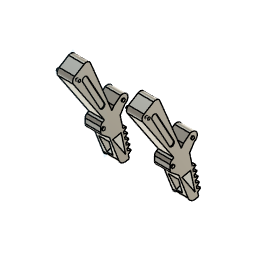
JAW FINAL v2 (Autodesk Fusion 360 design; units mm, degrees)
Autodesk Fusion 360 part; units mm, degrees
sketch "Sketch1" plane through (0, 0, 0) normal (1, 0, 0) x (0, 1, 0)
  line L0 (308.6071, 26.1218) -> (329.0653, 38.6702)
  line L1 (329.0653, 38.6702) -> (356.1703, -26.9523)
  line L2 (364.0358, -80.7741) -> (365.4972, -87.6198)
  line L3 (365.4972, -87.6198) -> (376.2548, -85.3234)
  line L4 (376.2548, -85.3234) -> (365.8164, -36.4251)
  line L5 (365.8164, -36.4251) -> (371.2115, -28.0053)
  line L6 (308.6071, 26.1218) -> (347.5605, -32.0386)
  line L7 (356.1703, -26.9523) -> (347.5605, -32.0386)
  line L8 (347.5605, -32.0386) -> (343.2556, -34.5818)
  line L9 (343.2556, -34.5818) -> (343.2556, -44.5818)
  line L10 (343.2556, -44.5818) -> (353.387, -52.7276)
  line L11 (343.2556, -44.5818) -> (352.5031, -44.5818) construction
  line L12 (353.387, -52.7276) -> (364.0358, -80.7741)
  line L13 (356.1703, -26.9523) -> (358.6771, -23.3241)
  line L14 (358.6771, -23.3241) -> (366.4246, -17.0014)
  arc A0 (371.2115, -28.0053) -> (363.9076, -19.0555) centre (368.8181, -22.5033) ccw
  dimension "d6" = 70
  dimension "d7" = 24
  dimension "d8" = 71
  dimension "d10" = 10
  dimension "d11" = 5
  dimension "d12" = 10
  dimension "d13" = 13
  dimension "d14" = 38.8
  dimension "d15" = 30
  dimension "d16" = 7
  dimension "d17" = 11
  dimension "d18" = 50
  dimension "d19" = 10
  dimension "d20" = 4.41
  dimension "d21" = 10
  dimension "d22" = 12
  constraint perpendicular L2 L3
  constraint perpendicular L3 L4
  constraint parallel L7 L8
  constraint vertical L9
  constraint horizontal L11
  constraint coincident L14.end A0
  constraint coincident L14 A0.end
  measures "d6" distance of L0.start L6.end
  measures "d7" distance of L0.start L0.end
  measures "d8" distance of L0.end L1.end
  measures "d10" distance of L1.end L6.end
  measures "d11" distance of L6.end L8.end
  measures "d12" distance of L8.end L9.end
  measures "d13" distance of L9.end L10.end
  measures "d14" angle of L10 L11
  measures "d15" distance of L2.start L10.end
  measures "d16" distance of L2.start L2.end
  measures "d17" distance of L2.end L3.end
  measures "d18" distance of L3.end L4.end
  measures "d19" distance of L4.end L5.end
  measures "d20" distance of L1.end L13.end
  measures "d21" distance of L13.end L14.end
  measures "d22" distance of L5.end L14.end
extrude "Extrude1" add sketch "Sketch1" along normal mid plane 18 contours L0 L1 L6 L7 | L2 L3 L4 L5 L7 L8 L9 L10 L12 L13 L14 A0 in component "Component"
sketch "Sketch2" plane through (-9, 0, 0) normal (-1, 0, 0) x (0, -1, 0)
  line L0 (-347.5605, -32.0386) -> (-308.6071, 26.1218)
  line L1 (-308.6071, 26.1218) -> (-329.0653, 38.6702)
  line L2 (-329.0653, 38.6702) -> (-356.1703, -26.9523)
  line L3 (-356.1703, -26.9523) -> (-358.6771, -23.3241)
  line L4 (-358.6771, -23.3241) -> (-366.4246, -17.0014)
  arc A0 (-366.4246, -17.0014) -> (-371.2115, -28.0053) centre (-368.8181, -22.5033) ccw
  line L5 (-371.2115, -28.0053) -> (-365.8164, -36.4251)
  line L6 (-365.8164, -36.4251) -> (-376.2548, -85.3234)
  line L7 (-376.2548, -85.3234) -> (-365.4972, -87.6198)
  line L8 (-365.4972, -87.6198) -> (-364.0358, -80.7741)
  line L9 (-364.0358, -80.7741) -> (-353.387, -52.7276)
  line L10 (-353.387, -52.7276) -> (-343.2556, -44.5818)
  line L11 (-343.2556, -44.5818) -> (-343.2556, -34.5818)
  line L12 (-343.2556, -34.5818) -> (-347.5605, -32.0386)
sketch "Sketch3" plane through (9, 0, 0) normal (1, 0, 0) x (0, 1, 0)
  line L0 (308.6071, 26.1218) -> (347.5605, -32.0386)
  line L1 (347.5605, -32.0386) -> (343.2556, -34.5818)
  line L2 (343.2556, -34.5818) -> (343.2556, -44.5818)
  line L3 (343.2556, -44.5818) -> (353.387, -52.7276)
  line L4 (353.387, -52.7276) -> (364.0358, -80.7741)
  line L5 (364.0358, -80.7741) -> (365.4972, -87.6198)
  line L6 (365.4972, -87.6198) -> (376.2548, -85.3234)
  line L7 (376.2548, -85.3234) -> (365.8164, -36.4251)
  line L8 (365.8164, -36.4251) -> (371.2115, -28.0053)
  arc A0 (371.2115, -28.0053) -> (366.4246, -17.0014) centre (368.8181, -22.5033) ccw
  line L9 (366.4246, -17.0014) -> (358.6771, -23.3241)
  line L10 (358.6771, -23.3241) -> (356.1703, -26.9523)
  line L11 (356.1703, -26.9523) -> (329.0653, 38.6702)
  line L12 (329.0653, 38.6702) -> (308.6071, 26.1218)
  line L13 (364.0358, -80.7741) -> (372.1529, -79.0413)
  line L14 (372.1529, -79.0413) -> (366.9337, -54.5922)
  line L15 (372.1529, -79.0413) -> (366.9337, -54.5922)
  line L16 (366.9337, -54.5922) -> (357.1541, -56.6798)
  line L17 (357.1541, -56.6798) -> (372.1529, -79.0413)
  dimension "d25" = 90
  dimension "d26" = 25
  dimension "d28" = 2.7
  dimension "d29" = 10
  constraint coincident L4.end L5.start
  constraint perpendicular L5 L13
  constraint perpendicular L14 L16
  measures "d25" angle of L13 L14
  measures "d26" distance of L13.end L14.end
  measures "d28" distance of L7 L15
  measures "d29" distance of L14.end L16.end
extrude "Extrude2" cut sketch "Sketch3" against normal blind 68 contours L14 L15 L16 L17 in component "Component"
sketch "Sketch4" plane through (9, 0, 0) normal (1, 0, 0) x (0, 1, 0)
  line L0 (366.9337, -54.5922) -> (372.1529, -79.0413)
  line L1 (372.1529, -79.0413) -> (357.1541, -56.6798)
  line L2 (357.1541, -56.6798) -> (366.9337, -54.5922)
  line L3 (308.6071, 26.1218) -> (347.5605, -32.0386)
  line L4 (347.5605, -32.0386) -> (343.2556, -34.5818)
  line L5 (343.2556, -34.5818) -> (343.2556, -44.5818)
  line L6 (343.2556, -44.5818) -> (353.387, -52.7276)
  line L7 (353.387, -52.7276) -> (364.0358, -80.7741)
  line L8 (364.0358, -80.7741) -> (365.4972, -87.6198)
  line L9 (365.4972, -87.6198) -> (376.2548, -85.3234)
  line L10 (376.2548, -85.3234) -> (365.8164, -36.4251)
  line L11 (365.8164, -36.4251) -> (371.2115, -28.0053)
  arc A0 (371.2115, -28.0053) -> (366.4246, -17.0014) centre (368.8181, -22.5033) ccw
  line L12 (366.4246, -17.0014) -> (358.6771, -23.3241)
  line L13 (358.6771, -23.3241) -> (356.1703, -26.9523)
  line L14 (356.1703, -26.9523) -> (329.0653, 38.6702)
  line L15 (329.0653, 38.6702) -> (308.6071, 26.1218)
  line L16 (376.2548, -85.3234) -> (375.2109, -80.4336)
  line L17 (375.2109, -80.4336) -> (374.3759, -76.5217)
  line L18 (374.7934, -78.4776) -> (378.7053, -77.6426)
  line L19 (378.7053, -77.6426) -> (374.3759, -76.5217)
  line L20 (375.2109, -80.4336) -> (378.7053, -77.6426)
  line L21 (373.854, -74.0768) -> (377.3483, -71.2858)
  line L22 (373.4364, -72.1208) -> (377.3483, -71.2858)
  line L23 (377.3483, -71.2858) -> (373.0189, -70.1649)
  line L24 (373.854, -74.0768) -> (373.0189, -70.1649)
  line L25 (372.497, -67.72) -> (375.9913, -64.929)
  line L26 (372.0794, -65.7641) -> (375.9913, -64.929)
  line L27 (375.9913, -64.929) -> (371.6619, -63.8081)
  line L28 (372.497, -67.72) -> (371.6619, -63.8081)
  line L29 (371.14, -61.3632) -> (374.6343, -58.5722)
  line L30 (370.7225, -59.4073) -> (374.6343, -58.5722)
  line L31 (374.6343, -58.5722) -> (370.3049, -57.4514)
  line L32 (371.14, -61.3632) -> (370.3049, -57.4514)
  line L33 (369.783, -55.0065) -> (373.2773, -52.2155)
  line L34 (369.3655, -53.0505) -> (373.2773, -52.2155)
  line L35 (373.2773, -52.2155) -> (368.9479, -51.0946)
  line L36 (369.783, -55.0065) -> (368.9479, -51.0946)
  dimension "d32" = 5
  dimension "d33" = 4
  dimension "d34" = 4
  dimension "d37" = 26
  dimension "d38" = 0
  constraint coincident L9.end L10.start
  constraint perpendicular L9 L16
  constraint perpendicular L9 L17
  constraint midpoint L17 L18.start
  constraint perpendicular L17 L18
  measures "d32" distance of L9.end L16.end
  measures "d33" distance of L16.end L17.end
  measures "d34" distance of L18.start L18.end
extrude "Extrude3" add sketch "Sketch4" against normal up to surface (18 mm away) contours L10 L34 L35 L36 | L10 L17 L18 L20 | L10 L33 L34 L36 | L10 L17 L18 L19 | L10 L30 L31 L32 | L10 L21 L22 L24 | L10 L29 L30 L32 | L10 L22 L23 L24 | L10 L26 L27 L28 | L10 L25 L26 L28 in component "Component"
fillet "Fillet1" radius 5 2 edges at (0, 308.6071, 26.1218) (0, 329.0653, 38.6702) in component "Component"
fillet "Fillet2" radius 7.5 1 edges at (0, 365.4972, -87.6198) in component "Component"
fillet "Fillet3" radius 4 2 edges at (0, 343.2556, -44.5818) (0, 343.2556, -34.5818) in component "Component"
sketch "Sketch5" plane through (9, 0, 0) normal (1, 0, 0) x (0, 1, 0)
  arc A0 (345.221, -33.4207) -> (343.2556, -36.8646) centre (347.2556, -36.8646) ccw
  line L0 (343.2556, -36.8646) -> (343.2556, -42.6653)
  arc A1 (343.2556, -42.6653) -> (344.7491, -45.7827) centre (347.2556, -42.6653) ccw
  line L1 (344.7491, -45.7827) -> (353.387, -52.7276)
  line L2 (353.387, -52.7276) -> (364.0358, -80.7741)
  arc A2 (364.0358, -80.7741) -> (372.8156, -86.0576) centre (371.2498, -78.7228) ccw
  line L3 (372.8156, -86.0576) -> (376.2548, -85.3234)
  line L4 (376.2548, -85.3234) -> (375.2109, -80.4336)
  line L5 (375.2109, -80.4336) -> (378.7053, -77.6426)
  line L6 (378.7053, -77.6426) -> (374.3759, -76.5217)
  line L7 (374.3759, -76.5217) -> (373.854, -74.0768)
  line L8 (373.854, -74.0768) -> (377.3483, -71.2858)
  line L9 (377.3483, -71.2858) -> (373.0189, -70.1649)
  line L10 (373.0189, -70.1649) -> (372.497, -67.72)
  line L11 (372.497, -67.72) -> (375.9913, -64.929)
  line L12 (375.9913, -64.929) -> (371.6619, -63.8081)
  line L13 (371.6619, -63.8081) -> (371.14, -61.3632)
  line L14 (371.14, -61.3632) -> (374.6343, -58.5722)
  line L15 (374.6343, -58.5722) -> (370.3049, -57.4514)
  line L16 (370.3049, -57.4514) -> (369.783, -55.0065)
  line L17 (369.783, -55.0065) -> (373.2773, -52.2155)
  line L18 (373.2773, -52.2155) -> (368.9479, -51.0946)
  line L19 (368.9479, -51.0946) -> (365.8164, -36.4251)
  line L20 (365.8164, -36.4251) -> (371.2115, -28.0053)
  arc A3 (371.2115, -28.0053) -> (366.4246, -17.0014) centre (368.8181, -22.5033) ccw
  line L21 (366.4246, -17.0014) -> (358.6771, -23.3241)
  line L22 (358.6771, -23.3241) -> (356.1703, -26.9523)
  line L23 (356.1703, -26.9523) -> (331.3034, 33.2516)
  arc A4 (331.3034, 33.2516) -> (324.0678, 35.6049) centre (326.6821, 31.3428) ccw
  line L24 (324.0678, 35.6049) -> (313.043, 28.8426)
  arc A5 (313.043, 28.8426) -> (311.5029, 21.7981) centre (315.6572, 24.5805) ccw
  line L25 (311.5029, 21.7981) -> (347.5605, -32.0386)
  line L26 (347.5605, -32.0386) -> (345.221, -33.4207)
  line L27 (366.9337, -54.5922) -> (372.1529, -79.0413)
  line L28 (372.1529, -79.0413) -> (357.1541, -56.6798)
  line L29 (357.1541, -56.6798) -> (366.9337, -54.5922)
  circle A6 centre (314.3303, 24.5805) radius 1.5
  dimension "d49" = 3
  measures "d49" diameter of A6
extrude "Extrude4" cut sketch "Sketch5" against normal blind 29 contours A6 in component "Component"
sketch "Sketch6" plane through (0, 291.3636, 110.6267) normal (0, -0.934881, -0.354961) x (1, 0, 0)
  line L0 (-9, -204.7328) -> (9, -204.7328)
  line L1 (9, -204.7328) -> (9, -174.7328)
  line L2 (9, -174.7328) -> (-9, -174.7328)
  line L3 (-9, -174.7328) -> (-9, -204.7328)
  line L4 (-6, -182.1738) -> (6, -182.1738)
  line L5 (-7, -201.7782) -> (3.528, -201.7782)
  line L6 (3.528, -201.7782) -> (6, -182.1738)
  line L7 (-6, -182.1738) -> (-3.4614, -201.7782)
  dimension "d52" = 3
  dimension "d53" = 3
  dimension "d54" = 7.441
  constraint horizontal L4
  constraint horizontal L5
  constraint coincident L5 L7.end
  measures "d52" distance of L1 L4.end
  measures "d53" distance of L3 L4.start
  measures "d54" distance of L2 L4
extrude "Extrude5" cut sketch "Sketch6" against normal blind 8 contours L4 L5 L6 L7 in component "Component"
sketch "Sketch7" plane through (9, 0, 0) normal (1, 0, 0) x (0, 1, 0)
  circle A0 centre (314.3303, 24.5805) radius 1.5
  arc A1 (345.221, -33.4207) -> (343.2556, -36.8646) centre (347.2556, -36.8646) ccw
  line L0 (343.2556, -36.8646) -> (343.2556, -42.6653)
  arc A2 (343.2556, -42.6653) -> (344.7491, -45.7827) centre (347.2556, -42.6653) ccw
  line L1 (344.7491, -45.7827) -> (353.387, -52.7276)
  line L2 (353.387, -52.7276) -> (364.0358, -80.7741)
  arc A3 (364.0358, -80.7741) -> (372.8156, -86.0576) centre (371.2498, -78.7228) ccw
  line L3 (372.8156, -86.0576) -> (376.2548, -85.3234)
  line L4 (376.2548, -85.3234) -> (375.2109, -80.4336)
  line L5 (375.2109, -80.4336) -> (378.7053, -77.6426)
  line L6 (378.7053, -77.6426) -> (374.3759, -76.5217)
  line L7 (374.3759, -76.5217) -> (373.854, -74.0768)
  line L8 (373.854, -74.0768) -> (377.3483, -71.2858)
  line L9 (377.3483, -71.2858) -> (373.0189, -70.1649)
  line L10 (373.0189, -70.1649) -> (372.497, -67.72)
  line L11 (372.497, -67.72) -> (375.9913, -64.929)
  line L12 (375.9913, -64.929) -> (371.6619, -63.8081)
  line L13 (371.6619, -63.8081) -> (371.14, -61.3632)
  line L14 (371.14, -61.3632) -> (374.6343, -58.5722)
  line L15 (374.6343, -58.5722) -> (370.3049, -57.4514)
  line L16 (370.3049, -57.4514) -> (369.783, -55.0065)
  line L17 (369.783, -55.0065) -> (373.2773, -52.2155)
  line L18 (373.2773, -52.2155) -> (368.9479, -51.0946)
  line L19 (368.9479, -51.0946) -> (365.8164, -36.4251)
  line L20 (365.8164, -36.4251) -> (371.2115, -28.0053)
  arc A4 (371.2115, -28.0053) -> (366.4246, -17.0014) centre (368.8181, -22.5033) ccw
  line L21 (366.4246, -17.0014) -> (358.6771, -23.3241)
  line L22 (358.6771, -23.3241) -> (356.1703, -26.9523)
  line L23 (356.1703, -26.9523) -> (331.3034, 33.2516)
  arc A5 (331.3034, 33.2516) -> (324.0678, 35.6049) centre (326.6821, 31.3428) ccw
  line L24 (324.0678, 35.6049) -> (313.043, 28.8426)
  arc A6 (313.043, 28.8426) -> (311.5029, 21.7981) centre (315.6572, 24.5805) ccw
  line L25 (311.5029, 21.7981) -> (347.5605, -32.0386)
  line L26 (347.5605, -32.0386) -> (345.221, -33.4207)
  line L27 (366.9337, -54.5922) -> (372.1529, -79.0413)
  line L28 (372.1529, -79.0413) -> (357.1541, -56.6798)
  line L29 (357.1541, -56.6798) -> (366.9337, -54.5922)
  circle A7 centre (368.8181, -22.5033) radius 1.75
  circle A8 centre (345.9618, -39.765) radius 1.75
  dimension "d57" = 3.5
  dimension "d58" = 3.5
  constraint concentric A4 A7
  measures "d57" diameter of A7
  measures "d58" diameter of A8
extrude "Extrude6" add sketch "Sketch7" along normal blind 1 contours A7 | A8 in component "Component"
sketch "Sketch8" plane through (9, 0, 0) normal (1, 0, 0) x (0, 1, 0)
  circle A0 centre (368.8181, -22.5033) radius 1.75
  circle A1 centre (345.9618, -39.765) radius 1.75
  circle A2 centre (314.3303, 24.5805) radius 1.5
  arc A3 (345.221, -33.4207) -> (343.2556, -36.8646) centre (347.2556, -36.8646) ccw
  line L0 (343.2556, -36.8646) -> (343.2556, -42.6653)
  arc A4 (343.2556, -42.6653) -> (344.7491, -45.7827) centre (347.2556, -42.6653) ccw
  line L1 (344.7491, -45.7827) -> (353.387, -52.7276)
  line L2 (353.387, -52.7276) -> (364.0358, -80.7741)
  arc A5 (364.0358, -80.7741) -> (372.8156, -86.0576) centre (371.2498, -78.7228) ccw
  line L3 (372.8156, -86.0576) -> (376.2548, -85.3234)
  line L4 (376.2548, -85.3234) -> (375.2109, -80.4336)
  line L5 (375.2109, -80.4336) -> (378.7053, -77.6426)
  line L6 (378.7053, -77.6426) -> (374.3759, -76.5217)
  line L7 (374.3759, -76.5217) -> (373.854, -74.0768)
  line L8 (373.854, -74.0768) -> (377.3483, -71.2858)
  line L9 (377.3483, -71.2858) -> (373.0189, -70.1649)
  line L10 (373.0189, -70.1649) -> (372.497, -67.72)
  line L11 (372.497, -67.72) -> (375.9913, -64.929)
  line L12 (375.9913, -64.929) -> (371.6619, -63.8081)
  line L13 (371.6619, -63.8081) -> (371.14, -61.3632)
  line L14 (371.14, -61.3632) -> (374.6343, -58.5722)
  line L15 (374.6343, -58.5722) -> (370.3049, -57.4514)
  line L16 (370.3049, -57.4514) -> (369.783, -55.0065)
  line L17 (369.783, -55.0065) -> (373.2773, -52.2155)
  line L18 (373.2773, -52.2155) -> (368.9479, -51.0946)
  line L19 (368.9479, -51.0946) -> (365.8164, -36.4251)
  line L20 (365.8164, -36.4251) -> (371.2115, -28.0053)
  arc A6 (371.2115, -28.0053) -> (366.4246, -17.0014) centre (368.8181, -22.5033) ccw
  line L21 (366.4246, -17.0014) -> (358.6771, -23.3241)
  line L22 (358.6771, -23.3241) -> (356.1703, -26.9523)
  line L23 (356.1703, -26.9523) -> (331.3034, 33.2516)
  arc A7 (331.3034, 33.2516) -> (324.0678, 35.6049) centre (326.6821, 31.3428) ccw
  line L24 (324.0678, 35.6049) -> (313.043, 28.8426)
  arc A8 (313.043, 28.8426) -> (311.5029, 21.7981) centre (315.6572, 24.5805) ccw
  line L25 (311.5029, 21.7981) -> (347.5605, -32.0386)
  line L26 (347.5605, -32.0386) -> (345.221, -33.4207)
  line L27 (366.9337, -54.5922) -> (372.1529, -79.0413)
  line L28 (372.1529, -79.0413) -> (357.1541, -56.6798)
  line L29 (357.1541, -56.6798) -> (366.9337, -54.5922)
  line L30 (322.3738, 18.5661) -> (342.5242, -18.3398)
  arc A9 (342.5242, -18.3398) -> (347.7767, -15.4719) centre (345.1504, -16.9058) ccw
  line L31 (347.7767, -15.4719) -> (327.6262, 21.4339)
  arc A10 (327.6262, 21.4339) -> (322.3738, 18.5661) centre (325, 20) ccw
  line L32 (325, 20) -> (345.1504, -16.9058) construction
  constraint tangent L30 A9
  constraint tangent A9 L31
  constraint parallel L30 L31
  constraint tangent L31 A10
  constraint tangent L30 A10
extrude "Extrude7" cut sketch "Sketch8" against normal blind 1 contours L30 A9 L31 A10 in component "Component"
mirror "Mirror1" about plane through (0, 344.5115, -25.3555) normal (1, 0, 0) of "Extrude6", "Extrude7" in component "Component"
sketch "Sketch9" plane through (9, 0, 0) normal (1, 0, 0) x (0, 1, 0)
  line L0 (342.5242, -18.3398) -> (322.3738, 18.5661)
  arc A0 (327.6262, 21.4339) -> (322.3738, 18.5661) centre (325, 20) ccw
  line L1 (327.6262, 21.4339) -> (347.7767, -15.4719)
  arc A1 (342.5242, -18.3398) -> (347.7767, -15.4719) centre (345.1504, -16.9058) ccw
  circle A2 centre (368.8181, -22.5033) radius 1.75
  circle A3 centre (345.9618, -39.765) radius 1.75
  circle A4 centre (314.3303, 24.5805) radius 1.5
  arc A5 (345.221, -33.4207) -> (343.2556, -36.8646) centre (347.2556, -36.8646) ccw
  line L2 (343.2556, -36.8646) -> (343.2556, -42.6653)
  arc A6 (343.2556, -42.6653) -> (344.7491, -45.7827) centre (347.2556, -42.6653) ccw
  line L3 (344.7491, -45.7827) -> (353.387, -52.7276)
  line L4 (353.387, -52.7276) -> (364.0358, -80.7741)
  arc A7 (364.0358, -80.7741) -> (372.8156, -86.0576) centre (371.2498, -78.7228) ccw
  line L5 (372.8156, -86.0576) -> (376.2548, -85.3234)
  line L6 (376.2548, -85.3234) -> (375.2109, -80.4336)
  line L7 (375.2109, -80.4336) -> (378.7053, -77.6426)
  line L8 (378.7053, -77.6426) -> (374.3759, -76.5217)
  line L9 (374.3759, -76.5217) -> (373.854, -74.0768)
  line L10 (373.854, -74.0768) -> (377.3483, -71.2858)
  line L11 (377.3483, -71.2858) -> (373.0189, -70.1649)
  line L12 (373.0189, -70.1649) -> (372.497, -67.72)
  line L13 (372.497, -67.72) -> (375.9913, -64.929)
  line L14 (375.9913, -64.929) -> (371.6619, -63.8081)
  line L15 (371.6619, -63.8081) -> (371.14, -61.3632)
  line L16 (371.14, -61.3632) -> (374.6343, -58.5722)
  line L17 (374.6343, -58.5722) -> (370.3049, -57.4514)
  line L18 (370.3049, -57.4514) -> (369.783, -55.0065)
  line L19 (369.783, -55.0065) -> (373.2773, -52.2155)
  line L20 (373.2773, -52.2155) -> (368.9479, -51.0946)
  line L21 (368.9479, -51.0946) -> (365.8164, -36.4251)
  line L22 (365.8164, -36.4251) -> (371.2115, -28.0053)
  arc A8 (371.2115, -28.0053) -> (366.4246, -17.0014) centre (368.8181, -22.5033) ccw
  line L23 (366.4246, -17.0014) -> (358.6771, -23.3241)
  line L24 (358.6771, -23.3241) -> (356.1703, -26.9523)
  line L25 (356.1703, -26.9523) -> (331.3034, 33.2516)
  arc A9 (331.3034, 33.2516) -> (324.0678, 35.6049) centre (326.6821, 31.3428) ccw
  line L26 (324.0678, 35.6049) -> (313.043, 28.8426)
  arc A10 (313.043, 28.8426) -> (311.5029, 21.7981) centre (315.6572, 24.5805) ccw
  line L27 (311.5029, 21.7981) -> (347.5605, -32.0386)
  line L28 (347.5605, -32.0386) -> (345.221, -33.4207)
  line L29 (366.9337, -54.5922) -> (372.1529, -79.0413)
  line L30 (372.1529, -79.0413) -> (357.1541, -56.6798)
  line L31 (357.1541, -56.6798) -> (366.9337, -54.5922)
  circle A11 centre (314.3303, 24.5805) radius 1.5
  constraint concentric A4 A11
extrude "Extrude8" add sketch "Sketch9" against normal blind 21 contours A4 A11 in component "Component"
sketch "Sketch10" plane through (9, 0, 0) normal (1, 0, 0) x (0, 1, 0)
  line L0 (342.5242, -18.3398) -> (322.3738, 18.5661)
  arc A0 (327.6262, 21.4339) -> (322.3738, 18.5661) centre (325, 20) ccw
  line L1 (327.6262, 21.4339) -> (347.7767, -15.4719)
  arc A1 (342.5242, -18.3398) -> (347.7767, -15.4719) centre (345.1504, -16.9058) ccw
  circle A2 centre (368.8181, -22.5033) radius 1.75
  circle A3 centre (345.9618, -39.765) radius 1.75
  arc A4 (345.221, -33.4207) -> (343.2556, -36.8646) centre (347.2556, -36.8646) ccw
  line L2 (343.2556, -36.8646) -> (343.2556, -42.6653)
  arc A5 (343.2556, -42.6653) -> (344.7491, -45.7827) centre (347.2556, -42.6653) ccw
  line L3 (344.7491, -45.7827) -> (353.387, -52.7276)
  line L4 (353.387, -52.7276) -> (364.0358, -80.7741)
  arc A6 (364.0358, -80.7741) -> (372.8156, -86.0576) centre (371.2498, -78.7228) ccw
  line L5 (372.8156, -86.0576) -> (376.2548, -85.3234)
  line L6 (376.2548, -85.3234) -> (375.2109, -80.4336)
  line L7 (375.2109, -80.4336) -> (378.7053, -77.6426)
  line L8 (378.7053, -77.6426) -> (374.3759, -76.5217)
  line L9 (374.3759, -76.5217) -> (373.854, -74.0768)
  line L10 (373.854, -74.0768) -> (377.3483, -71.2858)
  line L11 (377.3483, -71.2858) -> (373.0189, -70.1649)
  line L12 (373.0189, -70.1649) -> (372.497, -67.72)
  line L13 (372.497, -67.72) -> (375.9913, -64.929)
  line L14 (375.9913, -64.929) -> (371.6619, -63.8081)
  line L15 (371.6619, -63.8081) -> (371.14, -61.3632)
  line L16 (371.14, -61.3632) -> (374.6343, -58.5722)
  line L17 (374.6343, -58.5722) -> (370.3049, -57.4514)
  line L18 (370.3049, -57.4514) -> (369.783, -55.0065)
  line L19 (369.783, -55.0065) -> (373.2773, -52.2155)
  line L20 (373.2773, -52.2155) -> (368.9479, -51.0946)
  line L21 (368.9479, -51.0946) -> (365.8164, -36.4251)
  line L22 (365.8164, -36.4251) -> (371.2115, -28.0053)
  arc A7 (371.2115, -28.0053) -> (366.4246, -17.0014) centre (368.8181, -22.5033) ccw
  line L23 (366.4246, -17.0014) -> (358.6771, -23.3241)
  line L24 (358.6771, -23.3241) -> (356.1703, -26.9523)
  line L25 (356.1703, -26.9523) -> (331.3034, 33.2516)
  arc A8 (331.3034, 33.2516) -> (324.0678, 35.6049) centre (326.6821, 31.3428) ccw
  line L26 (324.0678, 35.6049) -> (313.043, 28.8426)
  arc A9 (313.043, 28.8426) -> (311.5029, 21.7981) centre (315.6572, 24.5805) ccw
  line L27 (311.5029, 21.7981) -> (347.5605, -32.0386)
  line L28 (347.5605, -32.0386) -> (345.221, -33.4207)
  line L29 (366.9337, -54.5922) -> (372.1529, -79.0413)
  line L30 (372.1529, -79.0413) -> (357.1541, -56.6798)
  line L31 (357.1541, -56.6798) -> (366.9337, -54.5922)
  circle A10 centre (315.6572, 24.5805) radius 1.5
  dimension "d67" = 3
  constraint concentric A9 A10
  measures "d67" diameter of A10
extrude "Extrude9" add sketch "Sketch10" along normal blind 3 contours A10 in component "Component"
sketch "Sketch11" plane through (-12, 0, 0) normal (-1, 0, 0) x (0, -1, 0)
  circle A0 centre (-314.3303, 24.5805) radius 1.5
component "Component" placed x (1, 0, 0) y (0, 1, 0) z (0, 0, 1) at (0, 0, 0)
component "Component" placed x (1, 0, 0) y (0, 1, 0) z (0, 0, 1) at (52.854, 27.602, -25.252)
